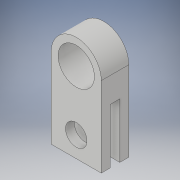
# Autodesk Inventor part: FrameMountingBracket
Saved by Autodesk Inventor 2019 (Build 230136000, 136)
## iProperties
Created: 2018-11-12
Part Number: FrameMountingBracket
Material: Generic
Document SubType Name: Modeling
Designer: steelen
Density: 1 g/cm^3
Appearance: Default
d0: 1.320 in
d1: 0.250 in
d7: 1.000 in
d8: 0.00 deg
d9: 0.781 in
d18: 0.350 in
d19: 0.325 in
d20: 2.000 in
d21: 0.00 deg
d23: 2.000 in
d24: 0.750 in
ArmOffsetDist: 2.160 in
Author: steelen
Autodesk Inventor part; units mm, degrees
ref_plane "YZ Plane" through (0, 0, 0) normal (1, 0, 0) x (0, 1, 0)
ref_plane "XZ Plane" through (0, 0, 0) normal (0, 1, 0) x (-1, 0, 0)
ref_plane "XY Plane" through (0, 0, 0) normal (0, 0, 1) x (1, 0, 0)
sketch "Sketch1" plane through (0, 0, 0) normal (0, 0, 1) x (1, 0, 0)
  circle A0 centre (0, 0) radius 16.764
  circle A1 centre (0, 0) radius 23.114
  line L0 (23.114, 0) -> (23.114, -73.914)
  line L1 (23.114, -73.914) -> (-23.114, -73.914)
  line L2 (-23.114, -73.914) -> (-23.114, 0)
  line L3 (23.114, -23.114) -> (0, -23.114)
  line L4 (-23.114, -23.114) -> (0, -23.114)
  dimension "d0" = 33.528
  dimension "d1" = 6.35
  dimension "d23" = 50.8
  constraints: 10 end point, 3 point on circle, 3 point on line, 3 tangent, 2 centre point, 2 coincident, 2 perpendicular, 1 collinear, 1 horizontal, 1 vertical
  measures "d0" diameter of A0
  measures "d1" radial gap between concentric circles of A1 A0
  measures "d23" distance between parallel lines of L4 L1
extrude "Extrusion2" add sketch "Sketch1" along normal blind 25.4
sketch "Sketch3" plane through (0, 0, 25.4) normal (0, 0, 1) x (1, 0, 0)
  line L0 (-23.114, 0) -> (-23.114, -73.914) projected
  line L1 (23.114, -73.914) -> (23.114, 0) projected
  line L2 (-23.114, -73.914) -> (23.114, -73.914)
  line L3 (23.114, -73.914) -> (23.114, -23.114)
  line L4 (23.114, -23.114) -> (-23.114, -23.114)
  line L5 (-23.114, -23.114) -> (-23.114, -73.914)
  arc A0 (23.114, 0) -> (-23.114, 0) centre (0, 0) ccw projected
  circle A1 centre (0, 0) radius 23.114
  line L6 (-23.114, -73.914) -> (23.114, -73.914) projected
  line L7 (0, -23.114) -> (0, -73.914)
  point P0 (0, -54.864)
  dimension "d24" = 19.05
  constraints: 10 end point, 2 horizontal, 2 midpoint, 2 parallel, 2 point on line, 1 coincident, 1 perpendicular, 1 vertical alignment, 3 other
  measures "d24" distance from line of L2 point (0, -54.864)
hole "Hole1" at (0, -54.864, 25.4) direction (0, 0, -1) diameter 19.8374 end through all clearance for "Hex Head Bolt" size "3/4" standard "Ansi Unified Screw Threads"
sketch "Sketch6" plane through (-23.114, -73.914, 0) normal (0, -1, 0) x (1, 0, 0)
  line L0 (46.228, 0) -> (46.228, 25.4) projected
  line L1 (0, 0) -> (0, 25.4) projected
  line L2 (46.228, 8.255) -> (0, 8.255)
  line L3 (0, 8.255) -> (0, 17.145)
  line L4 (0, 17.145) -> (46.228, 17.145)
  line L5 (46.228, 17.145) -> (46.228, 8.255)
  line L6 (46.228, 25.4) -> (0, 25.4) projected
  line L7 (46.228, 0) -> (0, 0) projected
  point P0 (23.114, 0)
  dimension "d18" = 8.89
  dimension "d19" = 8.255
  constraints: 8 end point, 2 parallel, 2 point on line, 1 horizontal, 1 perpendicular
  measures "d18" distance between parallel lines of L4 L2
  measures "d19" distance between parallel lines of L7 L2
extrude "Extrusion3" cut sketch "Sketch6" against normal blind 50.8 contours L2 L1 L4 L0
sketch "Sketch7" plane through (0, 0, 25.4) normal (0, 0, 1) x (1, 0, 0)
  circle A0 centre (0, -54.864) radius 9.9187 projected
  circle A1 centre (0, 0) radius 16.764 projected
  dimension "d25" = 54.864
  measures "d25" distance of A0.centre point (0, 0)
equation "\"d23\" = MountingArmLength"
equation "\"d19\" = ArmWidth"
equation "\"d20\" = MountingArmLength"
equation "\"ArmWidth\" = -0.5 * d18 + 0.5 * d7"
equation "\"ArmOffsetDist\" = d25"
equation "\"MountingArmLength\" = 50.8"
equation "\"d7\" = 25.4"
body "Solid2"
